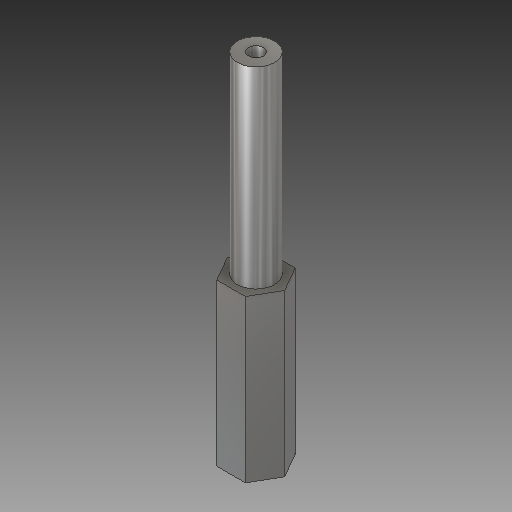
# Autodesk Inventor part: Roller drive shaft
Saved by Autodesk Inventor 2017 SP1 (Build 210196100, 196)
## iProperties
Created: 2018-02-02
Part Number: Roller drive shaft
Material: Generic
Document SubType Name: Modeling
Designer: Ben
Density: 1 g/cm^3
Appearance: Chrome - Polished
Mass: 8.24038 g
Surface Area: 46.2812 cm^2
Volume: 8.24038 cm^3
Author: Ben
Autodesk Inventor part; units mm, degrees
ref_plane "YZ Plane" through (0, 0, 0) normal (1, 0, 0) x (0, 1, 0)
ref_plane "XZ Plane" through (0, 0, 0) normal (0, 1, 0) x (-1, 0, 0)
ref_plane "XY Plane" through (0, 0, 0) normal (0, 0, 1) x (1, 0, 0)
sketch "Sketch1" plane through (0, 0, 0) normal (0, 1, 0) x (-1, 0, 0)
  line L0 (3.6662, -6.35) -> (-3.6662, -6.35)
  line L1 (-3.6662, -6.35) -> (-7.3323, 0)
  line L2 (-7.3323, 0) -> (-3.6662, 6.35)
  line L3 (-3.6662, 6.35) -> (3.6662, 6.35)
  line L4 (3.6662, 6.35) -> (7.3323, 0)
  line L5 (7.3323, 0) -> (3.6662, -6.35)
  circle A0 centre (0, 0) radius 1.905
  dimension "d0" = 12.7
  dimension "d6" = 3.81
  constraints: 12 end point, 2 coincident, 1 centre point, 1 horizontal, 13 other
  measures "d0" distance between parallel lines of L3 L0
  measures "d6" diameter of A0
extrude "Extrusion1" add sketch "Sketch1" against normal blind 41.275
sketch "Sketch2" plane through (0, 0, 0) normal (0, 1, 0) x (1, 0, 0)
  circle A0 centre (0, 0) radius 4.7625
  circle A1 centre (0, 0) radius 1.905 projected
  dimension "d3" = 9.525
  constraints: 1 centre point, 1 coincident
  measures "d3" diameter of A0
extrude "Extrusion2" add sketch "Sketch2" along normal blind 49.2125
body "Solid1"
